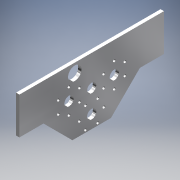
# Autodesk Inventor part: Inner Plate
Saved by Autodesk Inventor 2019.4 (Build 234330000, 330)
## iProperties
Created: 2019-12-07
Part Number: Inner Plate
Material: Aluminum 6061
Document SubType Name: Modeling
Designer: admin
Density: 2.7 g/cm^3
Appearance: Aluminum - Flat
Mass: 453.945 g
Surface Area: 568.361 cm^2
Volume: 168.128 cm^3
Author: admin
Autodesk Inventor part; units mm, degrees
ref_plane "YZ Plane" through (0, 0, 0) normal (1, 0, 0) x (0, 1, 0)
ref_plane "XZ Plane" through (0, 0, 0) normal (0, 1, 0) x (-1, 0, 0)
ref_plane "XY Plane" through (0, 0, 0) normal (0, 0, 1) x (1, 0, 0)
sketch "Sketch1" plane through (0, 0, 0) normal (1, 0, 0) x (0, 1, 0)
  line L0 (77, -100) -> (0, -100)
  line L1 (0, -100) -> (0, 100)
  line L2 (0, 100) -> (77, 100)
  line L3 (77, 100) -> (77, -100)
  line L4 (30, -90) -> (30, 90) construction
  line L5 (30, 0) -> (95.4693, 0) construction
  line L6 (60, -40) -> (-60, -40)
  line L7 (-60, -40) -> (-60, 40)
  line L8 (-60, 40) -> (60, 40)
  line L9 (60, 40) -> (60, -40)
  line L10 (60, -40) -> (-60, 40) construction
  line L11 (-60, -40) -> (60, 40) construction
  line L12 (-60, -40) -> (0, -100)
  line L13 (-60, -40) -> (24.8528, -40) construction
  line L14 (-60, 40) -> (0, 100)
  point P0 (0, 0)
  point P1 (0, 0)
  point P2 (0, 0)
  dimension "d2" = 77
  dimension "d3" = 200
  dimension "d7" = 180
  dimension "d8" = 30
  dimension "d9" = 100
  dimension "d10" = 120
  dimension "d11" = 80
  dimension "d12" = 45
  dimension "d13" = 45
  constraints: 30 end point, 5 midpoint, 4 horizontal, 4 parallel, 2 perpendicular, 2 point on line, 1 coincident, 1 equal length, 1 vertical
  measures "d2" distance of L0.start L0.end
  measures "d3" distance of L2.end L0.start
  measures "d7" distance of L4.end L4.start
  measures "d8" distance between parallel lines of L1 L4
  measures "d9" distance between parallel lines of L0 L5
  measures "d10" distance of L7.end L8.end
  measures "d11" distance of L6.end L7.end
  measures "d12" angle of L12 L13
  measures "d13" angle of L8 L14
extrude "Extrusion1" add sketch "Sketch1" along normal blind 7
sketch "Sketch2" plane through (7, 0, 0) normal (1, 0, 0) x (0, 0, -1)
  circle A0 centre (0, 14) radius 9.5
  circle A1 centre (0, 14) radius 40.64 construction
  circle A2 centre (-46.99, 14) radius 6.35 construction
  circle A3 centre (0, -32.99) radius 6.35 construction
  circle A4 centre (46.99, 14) radius 6.35 construction
  line L0 (0, 0) -> (0, 40) construction
  line L1 (100, 77) -> (-100, 77) projected
  circle A5 centre (0, -32.99) radius 9.65
  circle A6 centre (-46.99, 14) radius 9.65
  circle A7 centre (46.99, 14) radius 9.65
  line L2 (0, 14) -> (-46.99, 14) construction
  line L3 (0, 14) -> (46.99, 14) construction
  circle A8 centre (0, -32.99) radius 25.4 construction
  circle A9 centre (12.7, -54.987) radius 2.75
  circle A10 centre (0, -32.99) radius 25.4 construction
  circle A11 centre (25.4, -32.99) radius 2.75
  circle A12 centre (0, -32.99) radius 25.4 construction
  circle A13 centre (12.7, -10.993) radius 2.75
  circle A14 centre (0, -32.99) radius 25.4 construction
  circle A15 centre (-12.7, -10.993) radius 2.75
  circle A16 centre (0, -32.99) radius 25.4 construction
  circle A17 centre (-25.4, -32.99) radius 2.75
  circle A18 centre (0, -32.99) radius 25.4 construction
  circle A19 centre (-12.7, -54.987) radius 2.75
  line L4 (0, -32.99) -> (0, -43.499)
  line L5 (0, -32.99) -> (-12.7, -54.987)
  circle A20 centre (46.99, 14) radius 25.4 construction
  circle A21 centre (46.99, -11.4) radius 2.75
  circle A22 centre (68.987, 1.3) radius 2.75
  circle A23 centre (68.987, 26.7) radius 2.75
  circle A24 centre (46.99, 39.4) radius 2.75
  circle A25 centre (24.993, 26.7) radius 2.75
  circle A26 centre (24.993, 1.3) radius 2.75
  line L6 (46.99, 14) -> (46.99, -36) construction
  line L7 (46.99, 14) -> (96.99, 14) construction
  circle A27 centre (-46.99, 14) radius 25.4 construction
  circle A28 centre (-46.99, -11.4) radius 2.75
  line L8 (-46.99, 14) -> (-46.99, -11.4)
  line L9 (-46.99, 14) -> (-21.59, 14) construction
  circle A29 centre (-24.993, 1.3) radius 2.75
  circle A30 centre (-24.993, 26.7) radius 2.75
  circle A31 centre (-46.99, 39.4) radius 2.75
  circle A32 centre (-68.987, 26.7) radius 2.75
  circle A33 centre (-68.987, 1.3) radius 2.75
  circle A34 centre (0, 14) radius 22.5 construction
  circle A35 centre (-35, 58.0348) radius 33.75 construction
  circle A36 centre (-35, 58.0348) radius 14
  dimension "d28" = 50.8
  dimension "d36" = 50.8
  dimension "d44" = 50.8
  dimension "d14" = 19
  dimension "d15" = 81.28
  dimension "d16" = 12.7
  dimension "d17" = 12.7
  dimension "d18" = 12.7
  dimension "d20" = 63
  dimension "d21" = 19.3
  dimension "d22" = 19.3
  dimension "d23" = 19.3
  dimension "d24" = 90
  dimension "d25" = 90
  dimension "d29" = 5.5
  dimension "d32" = 360
  dimension "d35" = 30
  dimension "d37" = 5.5
  dimension "d40" = 360
  dimension "d42" = 50
  dimension "d43" = 90
  dimension "d45" = 5.5
  dimension "d46" = 90
  dimension "d49" = 360
  dimension "d52" = 45
  dimension "d53" = 67.5
  dimension "d54" = 35
  dimension "d55" = 28
  constraints: 29 centre point, 18 end point, 9 coincident, 4 tangent, 4 vertical, 3 point on line, 2 horizontal, 2 horizontal alignment, 2 perpendicular, 2 vertical alignment, 71 other
  measures "d14" diameter of A0
  measures "d15" diameter of A1
  measures "d16" diameter of A2
  measures "d17" diameter of A3
  measures "d18" diameter of A4
  measures "d20" distance from line of L1 A0.centre
  measures "d21" diameter of A5
  measures "d22" diameter of A6
  measures "d23" diameter of A7
  measures "d24" angle of L0 L2
  measures "d25" angle of L0 L3
  measures "d29" diameter of A9
  measures "d35" angle of L4 L5
  measures "d37" diameter of A21
  measures "d42" distance of L6.start L6.end
  measures "d43" angle of L6 L7
  measures "d45" diameter of A28
  measures "d46" angle of L8 L9
  measures "d52" diameter of A34
  measures "d53" diameter of A35
  measures "d54" distance from line of L0 A35.centre
  measures "d55" diameter of A36
extrude "Extrusion2" cut sketch "Sketch2" against normal blind 10
sketch "Sketch3" plane through (7, 0, 0) normal (1, 0, 0) x (0, 0, -1)
  line L0 (100, 77) -> (-100, 77) projected
  line L1 (100, 77) -> (600, 77)
  line L2 (600, 77) -> (600, 0)
  line L3 (600, 0) -> (100, 0)
  line L4 (100, 0) -> (100, 77)
  point P0 (0, 0)
  dimension "d56" = 500
  dimension "d57" = 77
  constraints: 8 end point, 2 parallel, 1 horizontal, 1 perpendicular
  measures "d56" distance of L2.end L3.end
  measures "d57" distance of L1.end L2.end
extrude "Extrusion3" add sketch "Sketch3" against normal blind 7
equation "\"d9\" = 0.5 * d3"
body "Solid1"
